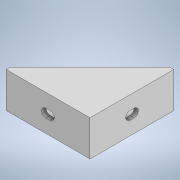
# Autodesk Inventor part: угол
Saved by Autodesk Inventor 2022 (Build 260153000, 153)
## iProperties
Created: 2022-04-26
Part Number: угол
Material: Типовые
Document SubType Name: Modeling
Designer: avkap
Density: 1 g/cm^3
Appearance: По умолчанию
Author: avkap
Autodesk Inventor part; units mm, degrees
ref_plane "YZ Plane" through (0, 0, 0) normal (1, 0, 0) x (0, 1, 0)
ref_plane "XZ Plane" through (0, 0, 0) normal (0, 1, 0) x (-1, 0, 0)
ref_plane "XY Plane" through (0, 0, 0) normal (0, 0, 1) x (1, 0, 0)
sketch "Эскиз1" plane through (0, 0, 0) normal (0, 1, 0) x (-1, 0, 0)
  line L0 (0, 0) -> (40, 0)
  line L1 (40, 0) -> (40, -40)
  line L2 (40, -40) -> (0, -40)
  line L3 (0, -40) -> (0, 0)
  line L4 (40, 0) -> (40, -2)
  line L5 (0, -40) -> (2, -40)
  line L6 (40, -2) -> (2, -40)
  dimension "d0" = 40
  dimension "d1" = 40
  dimension "d2" = 2
  dimension "d3" = 2
  constraints: 14 end point, 2 parallel, 2 point on line, 1 horizontal, 1 perpendicular
  measures "d0" distance of L1.end L2.end
  measures "d1" distance of L0.end L1.end
  measures "d2" distance of L0.end L4.end
  measures "d3" distance of L2.end L5.end
extrude "Выдавливание1" add sketch "Эскиз1" along normal blind 17 contours L0 L1 L6 L2 L3
sketch "Эскиз2" plane through (0, 0, -40) normal (0, 0, -1) x (-1, 0, 0)
  line L0 (0, 17) -> (2, 17) projected
  line L1 (2, 17) -> (2, 15)
  line L2 (2, 0) -> (2, 17) projected
  line L3 (2, 15) -> (40, 15)
  line L4 (40, 0) -> (40, 17) projected
  line L5 (0, 0) -> (2, 0) projected
  line L6 (2, 0) -> (2, 2)
  line L7 (2, 2) -> (40, 2)
  line L8 (40, 2) -> (40, 15)
  line L9 (2, 15) -> (2, 2)
  dimension "d6" = 2
  dimension "d7" = 2
  constraints: 12 end point, 3 point on line, 2 perpendicular, 1 collinear, 1 horizontal
  measures "d6" distance of L0.end L1.end
  measures "d7" distance of L2.start L6.end
extrude "Выдавливание2" cut sketch "Эскиз2" against normal blind 38
sketch "Эскиз3" plane through (0, 0, -2) normal (0, 0, -1) x (-1, 0, 0)
  line L0 (0, 0) -> (0, 17) projected
  line L1 (20, 10.2321) -> (20, 10.5)
  line L2 (20, 10.5) -> (21, 10.5)
  line L3 (21, 6.5) -> (19, 6.5)
  line L4 (19, 10.5) -> (20, 10.5)
  arc A0 (21, 6.5) -> (21, 10.5) centre (21, 8.5) ccw
  arc A1 (19, 10.5) -> (19, 6.5) centre (19, 8.5) ccw
  line L5 (20, 10.5) -> (20, 8.5)
  line L6 (0, 8.5) -> (17, 8.5)
  line L7 (19, 8.5) -> (20, 8.5)
  dimension "d10" = 20
  dimension "d11" = 2
  dimension "d13" = 1
  constraints: 14 end point, 5 point on circle, 3 perpendicular, 2 centre point, 2 horizontal, 2 point on line, 1 midpoint
  measures "d10" distance of L6.start L5.end
  measures "d11" distance of L5.end L1.end
  measures "d13" distance of L2.end L1.end
extrude "Выдавливание3" cut sketch "Эскиз3" against normal blind 10
sketch "Эскиз4" plane through (-2, 2, -40) normal (-1, 0, 0) x (0, 0, 1)
  line L0 (0, 0) -> (0, 13) projected
  line L1 (0, 6.5) -> (20, 6.5)
  line L2 (20, 8.2321) -> (20, 8.5)
  line L3 (20, 8.5) -> (21, 8.5)
  line L4 (21, 4.5) -> (20, 4.5)
  line L5 (20, 4.5) -> (19, 4.5)
  line L6 (19, 8.5) -> (20, 8.5)
  arc A0 (21, 4.5) -> (21, 8.5) centre (21, 6.5) ccw
  arc A1 (19, 8.5) -> (19, 4.5) centre (19, 6.5) ccw
  point P0 (40, -2)
  dimension "d17" = 20
  constraints: 12 end point, 5 point on circle, 3 point on line, 2 centre point, 1 horizontal, 1 midpoint, 1 perpendicular, 1 vertical
  measures "d17" distance of L1.start L1.end
extrude "Выдавливание5" cut sketch "Эскиз4" against normal blind 18.75
